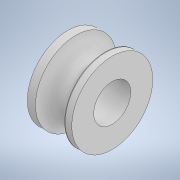
# Autodesk Inventor part: Riemenadapter
Saved by Autodesk Inventor 2021 (Build 250183000, 183)
## iProperties
Created: 2022-06-27
Part Number: Riemenadapter
Material: Generisch
Document SubType Name: Modeling
Designer: adria
Density: 1 g/cm^3
Appearance: Vorgabe
Mass: 2.13804 g
Surface Area: 19.1141 cm^2
Volume: 2.13804 cm^3
Author: adria
Autodesk Inventor part; units mm, degrees
ref_plane "YZ Plane" through (0, 0, 0) normal (1, 0, 0) x (0, 1, 0)
ref_plane "XZ Plane" through (0, 0, 0) normal (0, 1, 0) x (-1, 0, 0)
ref_plane "XY Plane" through (0, 0, 0) normal (0, 0, 1) x (1, 0, 0)
sketch "Skizze1" plane through (0, 0, 0) normal (0, 0, 1) x (1, 0, 0)
  line L0 (-6.1139, 5) -> (-6.1139, 10.9187)
  line L1 (-6.1139, 10.9187) -> (-3.9014, 10.9187)
  arc A0 (-3.9014, 10.9187) -> (3.9685, 10.9187) centre (0.0336, 10.9187) ccw
  arc A1 (3.9685, 10.9187) -> (4.1124, 10.9187) centre (4.0404, 10.9187) ccw
  line L2 (4.1124, 10.9187) -> (5.8861, 10.9187)
  line L3 (5.8861, 10.9187) -> (5.8861, 5)
  line L4 (5.8861, 5) -> (-6.1139, 5)
  line L5 (0, -2.1837) -> (0, 13.1025) projected
  line L6 (-8.5139, 0) -> (8.2861, 0) projected
  point P0 (0, 0)
  dimension "d0" = 5
  dimension "d1" = 12
  constraints: 10 end point, 4 point on circle, 3 point on line, 2 centre point, 2 horizontal, 2 vertical, 1 tangent
  measures "d0" distance from line of point (0, 0) L4
  measures "d1" distance between parallel lines of L0 L3
revolve "Umdrehung1" add sketch "Skizze1" angle 360 about axis through (-10, 0, 0) along (1, 0, 0)
